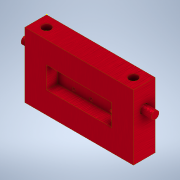
# Autodesk Inventor part: middle part edited
Saved by Autodesk Inventor 2021.3 (Build 253353000, 353)
## iProperties
Created: 2021-07-03
Part Number: middle part edited
Material: Polyethylene, High Density
Document SubType Name: Modeling
Designer: ASUS
Density: 0.952 g/cm^3
Appearance: Smooth - Off-White
Author: ASUS
Autodesk Inventor part; units mm, degrees
ref_plane "YZ Plane" through (0, 0, 0) normal (1, 0, 0) x (0, 1, 0)
ref_plane "XZ Plane" through (0, 0, 0) normal (0, 1, 0) x (-1, 0, 0)
ref_plane "XY Plane" through (0, 0, 0) normal (0, 0, 1) x (1, 0, 0)
sketch "Sketch1" plane through (0, 0, 0) normal (0, 0, 1) x (1, 0, 0)
  line L0 (0, 60) -> (0, 0)
  line L1 (0, 0) -> (100, 0)
  line L2 (100, 0) -> (100, 60)
  line L3 (100, 60) -> (0, 60)
  dimension "d0" = 100
  dimension "d1" = 60
  constraints: 8 end point, 3 perpendicular, 1 vertical
  measures "d0" distance of L1.end L0.end
  measures "d1" distance of L1.end L2.end
extrude "Extrusion1" add sketch "Sketch1" along normal blind 20
sketch "Sketch2" plane through (0, 0, 20) normal (0, 0, 1) x (1, 0, 0)
  line L0 (20, 40) -> (80, 40)
  line L1 (80, 40) -> (80, 20)
  line L2 (80, 20) -> (20, 20)
  line L3 (20, 20) -> (20, 40)
  line L4 (0, 60) -> (0, 0) projected
  line L5 (100, 0) -> (100, 60) projected
  line L6 (100, 60) -> (0, 60) projected
  line L7 (0, 0) -> (100, 0) projected
  dimension "d4" = 20
  dimension "d5" = 20
  dimension "d6" = 20
  dimension "d7" = 20
  dimension "d8" = 60
  dimension "d9" = 20
  constraints: 8 end point, 2 parallel, 1 horizontal, 1 perpendicular
  measures "d4" distance from line of L4 L2.end
  measures "d5" distance between parallel lines of L5 L1
  measures "d6" distance between parallel lines of L6 L0
  measures "d7" distance between parallel lines of L7 L2
  measures "d8" distance of L1.end L2.end
  measures "d9" distance of L1.end L0.end
extrude "Extrusion2" cut sketch "Sketch2" against normal blind 10 contours L0 L1 L2 L3
sketch "Sketch3" plane through (100, 0, 0) normal (1, 0, 0) x (0, 0, -1)
  circle A0 centre (-10, 40) radius 4
  point P0 (0, 0)
  dimension "d12" = 8
  constraints: 1 centre point
  measures "d12" diameter of A0
extrude "Extrusion3" cut sketch "Sketch3" against normal through all
sketch "Sketch4" plane through (0, 60, 0) normal (0, 1, 0) x (1, 0, 0)
  line L0 (100, 0) -> (0, 0) projected
  line L1 (100, -20) -> (0, -20) projected
  line L2 (100, 0) -> (100, -20) projected
  line L3 (0, 0) -> (100, 0) projected
  line L4 (0, 0) -> (0, -20) projected
  line L5 (100, -6) -> (100, -14) projected
  circle A0 centre (10, -10) radius 4
  circle A1 centre (90, -10) radius 4
  dimension "d21" = 20
  dimension "d27" = 8
  dimension "d28" = 8
  dimension "d29" = 80
  constraints: 2 centre point
  measures "d21" distance between parallel lines of L1 L0
  measures "d27" diameter of A0
  measures "d28" diameter of A1
  measures "d29" distance of A1.centre A0.centre
sketch "Sketch5" plane through (0, 60, 0) normal (0, 1, 0) x (1, 0, 0)
  point P0 (0, 0)
extrude "Extrusion4" cut sketch "Sketch4" against normal blind 5 contours A0 | A1
sketch "Sketch6" plane through (0, 0, 0) normal (0, -1, 0) x (1, 0, 0)
  circle A0 centre (10, 10) radius 4 projected
  circle A1 centre (10, 10) radius 4
  circle A2 centre (90, 10) radius 4 projected
  circle A3 centre (90, 10) radius 4
  line L0 (0, 0) -> (0, 20) projected
  line L1 (100, 0) -> (100, 20) projected
  dimension "d32" = 8
  dimension "d33" = 8
  dimension "d34" = 80
  dimension "d35" = 10
  dimension "d36" = 10
  constraints: 2 centre point, 2 coincident
  measures "d32" diameter of A1
  measures "d33" diameter of A3
  measures "d34" distance of A3.centre A1.centre
  measures "d35" distance from line of L0 A1.centre
  measures "d36" distance from line of L1 A3.centre
extrude "Extrusion5" cut sketch "Sketch6" against normal blind 5
sketch "Sketch7" plane through (0, 0, 20) normal (0, 0, 1) x (1, 0, 0)
  circle A0 centre (34.9582, 22.8628) radius 1.5
  circle A1 centre (50.8899, 22.8628) radius 1.5
  circle A2 centre (69.8112, 22.8628) radius 1.5
  point P0 (0, 0)
  dimension "d39" = 3
  dimension "d40" = 3
  dimension "d41" = 3
  constraints: 3 centre point
  measures "d39" diameter of A0
  measures "d40" diameter of A1
  measures "d41" diameter of A2
extrude "Extrusion6" cut sketch "Sketch7" against normal through all
sketch "Sketch8" plane through (0, 0, 0) normal (0, 0, -1) x (-1, 0, 0)
  line L0 (-77.8976, 17.9584) -> (-26.2908, 17.9584)
  line L1 (-26.2908, 17.9584) -> (-26.2908, 4.1966)
  line L2 (-26.2908, 4.1966) -> (-77.8976, 4.1966)
  line L3 (-77.8976, 4.1966) -> (-77.8976, 17.9584)
  point P0 (0, 0)
  constraints: 8 end point, 2 parallel, 1 horizontal, 1 perpendicular
extrude "Extrusion7" cut sketch "Sketch8" against normal blind 5
sketch "Sketch9" plane through (26.2908, 17.9584, 0) normal (0, -1, 0) x (1, 0, 0)
  circle A0 centre (44.1597, 2.2353) radius 1.5
  circle A1 centre (25.1097, 2.2353) radius 1.5
  circle A2 centre (8.9126, 2.2353) radius 1.5
  point P0 (-26.2908, 0)
  dimension "d46" = 3
  dimension "d47" = 3
  dimension "d48" = 3
  constraints: 3 centre point
  measures "d46" diameter of A0
  measures "d47" diameter of A1
  measures "d48" diameter of A2
extrude "Extrusion8" cut sketch "Sketch9" against normal blind 5
sketch "Sketch10" plane through (0, 0, 0) normal (0, -1, 0) x (1, 0, 0)
  point P0 (0, 0)
sketch "Sketch11" plane through (100, 0, 0) normal (1, 0, 0) x (0, 0, -1)
  circle A0 centre (-10, 40) radius 4 projected
  circle A1 centre (-10, 40) radius 3.5
  point P0 (0, 0)
  dimension "d51" = 7
  constraints: 1 centre point, 1 coincident
  measures "d51" diameter of A1
extrude "Extrusion9" add sketch "Sketch11" along normal mid plane 20 contours A1
sketch "Sketch12" plane through (0, 0, 0) normal (-1, 0, 0) x (0, 0, 1)
  circle A0 centre (10, 40) radius 3.5 projected
  circle A1 centre (10, 40) radius 3.5
  point P0 (0, 0)
  constraints: 1 centre point, 1 coincident
extrude "Extrusion10" add sketch "Sketch12" along normal mid plane 20
body "Solid1"
